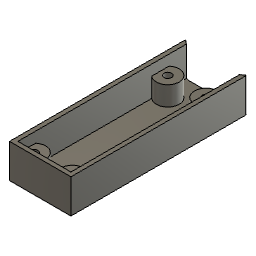
MB-RL7021-11-M5StickC Upper v6 (Autodesk Fusion 360 design; units mm, degrees)
Autodesk Fusion 360 part; units mm, degrees
sketch "スケッチ3" plane through (0, 0, 0) normal (0, 1, 0) x (1, 0, 0)
  line L0 (0, 0) -> (24.15, 0)
  line L1 (24.15, 0) -> (24.15, -67.65)
  line L2 (24.15, -67.65) -> (0, -67.65)
  line L3 (0, -67.65) -> (0, 0)
  arc A0 (21.15, 0) -> (23.7006, 1.2675) centre (21.15, 3.2) ccw
  line L4 (21.15, 3.2) -> (21.15, 0) construction
  line L5 (21.15, 3.2) -> (23.7006, 1.2675) construction
  line L6 (24.15, 0) -> (24.15, 1.12)
  arc A1 (24.15, 1.12) -> (23.7006, 1.2675) centre (23.9011, 1.12) ccw
  line L7 (22.5, -67.65) -> (22.5, 0.2987)
  line L8 (0, -66) -> (24, -66)
  circle A2 centre (19.575, -10) radius 1.5
  line L9 (12.075, -67.65) -> (12.075, 0)
  circle A3 centre (19.575, -62.5) radius 1.5
  arc A4 (0.4494, 1.2675) -> (3, 0) centre (3, 3.2) ccw
  line L10 (0, 0) -> (0, 1.12)
  arc A5 (0.4494, 1.2675) -> (0, 1.12) centre (0.2489, 1.12) ccw
  line L11 (1.65, -67.65) -> (1.65, 0.2987)
  circle A6 centre (4.575, -62.5) radius 1.5
  circle A7 centre (4.575, -10) radius 1.5
  circle A8 centre (6.575, -46.5) radius 1
  circle A9 centre (19.575, -62.5) radius 4.5
  circle A10 centre (19.575, -10) radius 4.5
  circle A11 centre (4.575, -62.5) radius 4.5
  circle A12 centre (4.575, -10) radius 4.5
  point P0 (21.15, 0)
  point P1 (21.15, 3.2)
  point P2 (23.9, 0.8469)
  dimension "d1" = 24.15
  dimension "d4" = 3.2
  dimension "d5" = 3
  dimension "d6" = 52.85
  dimension "d10" = 1.12
  dimension "d12" = 1.65
  dimension "d13" = 1.65
  dimension "d14" = 3
  dimension "d15" = 10
  dimension "d16" = 12.075
  dimension "d17" = 7.5
  dimension "d18" = 3
  dimension "d19" = 62.5
  dimension "d20" = 66
  dimension "d21" = 2
  dimension "d22" = 5.5
  dimension "d23" = 46.5
  dimension "d31" = 9
  dimension "d32" = 9
  dimension "d33" = 7.5
  constraint horizontal L0
  constraint vertical L1
  constraint horizontal L2
  constraint vertical L3
  constraint coincident L0.start L3.end
  constraint coincident L0 P0
  constraint coincident P0 A0.start
  constraint coincident P1 A0.centre
  constraint perpendicular L0 L6
  constraint tangent L6 A1
  constraint coincident L2 L7.start
  constraint coincident A0 L7.end
  constraint perpendicular L0 L7
  constraint coincident L3 L8.start
  constraint perpendicular L7 L8
  constraint coincident L2 L9.start
  constraint coincident L0 L9.end
  constraint perpendicular L0 L9
  constraint symmetric L0.end L9 L0.start
  constraint symmetric P0 L9 A4.end
  constraint symmetric A0.end L9 A4.start
  constraint symmetric A0 L9 A4
  constraint symmetric L6.end L9 L10.end
  constraint symmetric A1 L9 A5
  constraint symmetric L7.start L9 L11.start
  constraint symmetric L7.end L9 L11.end
  constraint symmetric A2 L9 A7
  constraint symmetric L9 A3 A6
  constraint concentric A3 A9
  constraint concentric A2 A10
  constraint symmetric L9 A9 A11
  constraint symmetric L9 A10 A12
  measures "d1" distance of L0.start L0.end
  measures "d4" distance of P0 P1
  measures "d5" distance of L0.end P0
  measures "d6" angle of L4 L5
  measures "d10" distance of L0.end L6.end
  measures "d12" distance of L1 L7
  measures "d13" distance of L2 L8
  measures "d14" diameter of A2
  measures "d15" distance of L0 A2.centre
  measures "d16" distance of L1 L9
  measures "d17" distance of A2.centre L9
  measures "d18" diameter of A3
  measures "d19" distance of L0 A3.centre
  measures "d20" distance of L0 L8
  measures "d21" diameter of A8
  measures "d22" distance of L9 A8.centre
  measures "d23" distance of L0 A8.centre
  measures "d31" diameter of A10
  measures "d32" diameter of A9
  measures "d33" distance of L9 A3.centre
extrude "押し出し1" add sketch "スケッチ3" along normal blind 13.35 contours L0 L8 L9 L11 A11 A12 | L0 A4 L11 | L0 L7 L8 L9 A9 A10 | L0 L3 L8 L11 A11 A12 | L0 A4 L10 A5 L11 | L0 A0 L7 | L2 L8 L9 L11 A11 | L2 L7 L8 L9 A9 | L11 A12 | L11 A12 | L0 A0 L6 A1 L7 | L0 L1 L2 L7 A9 A10 | L8 A11 | L8 L11 A11 | L7 L8 A9 | L8 A9 | L2 L3 L8 L11 | L7 A10 | L7 A10 | L8 L11 A11 | L7 L8 A9 | L7 A9 | L11 A11 | A2 | A3 | A6 | A7 | A8
extrude "押し出し3" cut sketch "スケッチ3" against normal blind 11.7 from surface at 13.35 contours L0 L8 L9 L11 A11 A12 | L0 A4 L11 | L0 L7 L8 L9 A9 A10 | L0 A0 L7 | L11 A12 | L8 L11 A11 | L7 L8 A9 | L7 A10 | L8 L11 A11 | L7 L8 A9 | A2 | A3 | A6 | A7 | A8 picked at (2.125, -10) picked at (22.025, -10)
extrude "押し出し4" add sketch "スケッチ3" along normal blind 9.25 contours L11 A12 | L8 A11 | L8 L11 A11 | L7 L8 A9 | L8 A9 | L7 A10 picked at (2.125, -10) picked at (4.6124, -65.3319) picked at (19.5376, -65.3319) picked at (22.025, -10)
extrude "押し出し5" add sketch "スケッチ3" along normal blind 2.75 contours A2 | A3 | A6 | A7
